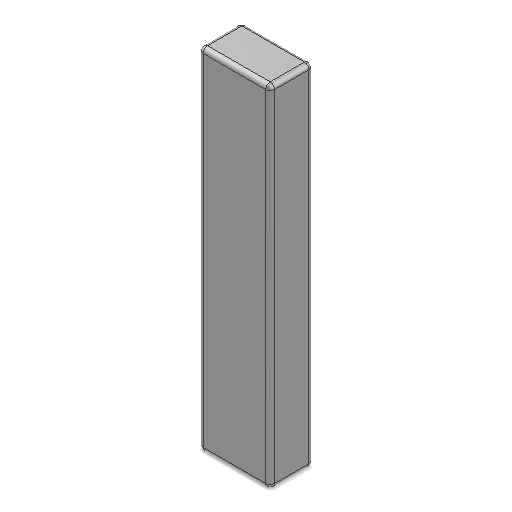
# Autodesk Inventor part: PSU
Saved by Autodesk Inventor 2026.2 (Build 302298000, 298)
## iProperties
Created: 2026-03-31
Part Number: PSU
Material: Aluminum 6061
Document SubType Name: Modeling
Designer: gaoet
Density: 2.7 g/cm^3
Appearance: Anodized - Light Gray
Author: gaoet
Autodesk Inventor part; units mm, degrees
ref_plane "YZ Plane" through (0, 0, 0) normal (1, 0, 0) x (0, 1, 0)
ref_plane "XZ Plane" through (0, 0, 0) normal (0, 1, 0) x (-1, 0, 0)
ref_plane "XY Plane" through (0, 0, 0) normal (0, 0, 1) x (1, 0, 0)
sketch "Sketch1" plane through (0, 0, 0) normal (0, 0, 1) x (1, 0, 0)
  line L0 (-24, -117.5) -> (24, -117.5)
  line L1 (24, -117.5) -> (24, 117.5)
  line L2 (24, 117.5) -> (-24, 117.5)
  line L3 (-24, 117.5) -> (-24, -117.5)
  line L4 (-24, -117.5) -> (24, 117.5) construction
  line L5 (24, -117.5) -> (-24, 117.5) construction
  point P0 (0, 0)
  dimension "d0" = 48
  dimension "d1" = 235
  constraints: 12 end point, 2 midpoint, 2 parallel, 1 horizontal, 1 perpendicular
  measures "d0" distance of L2.end L1.end
  measures "d1" distance of L1.end L0.end
extrude "Extrusion1" add sketch "Sketch1" along normal blind 29
fillet "Fillet1" radius 3 12 edges at (24, 0, 29) (24, 0, 0) (24, 117.5, 14.5) (0, 117.5, 29) (0, 117.5, 0) (-24, 117.5, 14.5) (-24, 0, 29) (-24, 0, 0) (-24, -117.5, 14.5) (0, -117.5, 29) (24, -117.5, 14.5) (0, -117.5, 0)
body "Solid1"
